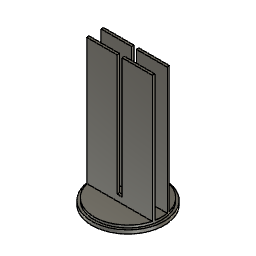
Can with 1 and 2 Vertical Shelves (Autodesk Fusion 360 design; units mm, degrees)
Autodesk Fusion 360 part; units mm, degrees
sketch "Base" plane through (0, 0, 0) normal (0, 0, 1) x (1, 0, 0)
  circle A0 centre (0, 0) radius 30
  circle A1 centre (0, 0) radius 28
  dimension "d1" = 60
  dimension "d2" = 56
  constraint coincident A0.centre A1.centre
  constraint concentric A0 A1
  measures "d1" diameter of A0
  measures "d2" diameter of A1
extrude "Extrude1" add sketch "Base" along normal blind 2 contours A1 makes body 1
extrude "Extrude2" add sketch "Base" along normal blind 113 bodies 1
sketch "Sketch2" plane through (0, 0, 0) normal (0, 0, 1) x (1, 0, 0)
  circle A0 centre (0, 0) radius 28
  line L0 (0, -2) -> (27.9285, -2)
  line L1 (-27.9285, -2) -> (0, -2)
  line L2 (0, 2) -> (-27.9285, 2)
  line L3 (27.9285, 2) -> (0, 2)
  circle A1 centre (0, 0) radius 30
  constraint coincident A0.centre A1.centre
  constraint coincident A0 L0.end
  constraint horizontal L0
  constraint coincident A0 L1.start
  constraint parallel L0 L1
  constraint coincident A0 L2.end
  constraint parallel L0 L2
  constraint coincident A0 L3.start
  constraint parallel L2 L3
extrude "Extrude3" add sketch "Sketch2" along normal blind 3 separate body makes body 2
extrude "Extrude4" add sketch "Sketch2" along normal blind 5 contours A0 L0 L1 bodies 2
extrude "Extrude5" add sketch "Sketch2" along normal blind 5 contours A0 L2 L3 bodies 2
extrude "Extrude6" add sketch "Sketch2" along normal blind 110 contours A0 L0 L1 L2 L3 bodies 2
sketch "Sketch6" plane through (0, 2, 0) normal (0, 1, 0) x (-1, 0, 0)
  line L0 (-27.9285, 5) -> (27.9285, 5)
  line L1 (27.9285, 5) -> (27.9285, 110)
  line L2 (27.9285, 110) -> (-27.9285, 110)
  line L3 (-27.9285, 110) -> (-27.9285, 5)
  line L4 (-2.5, 7.5) -> (2.5, 7.5)
  line L5 (2.5, 7.5) -> (2.5, 110)
  line L6 (-2.5, 110) -> (2.5, 110)
  line L7 (-2.5, 110) -> (-2.5, 7.5)
  dimension "d15" = 102.5
  dimension "d16" = 5
  constraint parallel L0 L4
  constraint coincident L2 L5.end
  constraint perpendicular L2 L5
  constraint coincident L2 L6.start
  constraint perpendicular L4 L7
  measures "d15" distance of L4.end L5.end
  measures "d16" distance of L5.end L6.start
extrude "Extrude7" cut sketch "Sketch6" against normal blind 4 contours L2 L4 L5 L6 L7 bodies 2
sketch "Sketch7" plane through (0, 0, 0) normal (0, 0, 1) x (1, 0, 0)
  circle A0 centre (-100, 0) radius 30
  circle A1 centre (-100, 0) radius 28
  line L0 (-100, 5) -> (-72.45, 5)
  line L1 (-100, -5) -> (-72.45, -5)
  line L2 (-100, -5) -> (-127.55, -5)
  line L3 (-100, 5) -> (-127.55, 5)
  line L4 (-100, -7) -> (-72.8891, -7)
  line L5 (-100, -7) -> (-127.1109, -7)
  line L6 (-100, 7) -> (-72.8891, 7)
  line L7 (-100, 7) -> (-127.1109, 7)
  constraint coincident A1 L0.end
  constraint coincident A1 L1.end
  constraint coincident A1 L2.end
  constraint coincident A1 L3.end
  constraint coincident A1 L4.end
  constraint parallel L2 L4
  constraint coincident A1 L5.end
  constraint parallel L4 L5
  constraint coincident A1 L6.end
  constraint horizontal L6
  constraint coincident A1 L7.end
  constraint parallel L6 L7
extrude "Extrude8" add sketch "Sketch7" along normal blind 3 separate body makes body 3
extrude "Extrude9" add sketch "Sketch7" along normal blind 5 contours A1 L6 L7 bodies 3
extrude "Extrude10" add sketch "Sketch7" along normal blind 5 contours A1 L0 L1 L2 L3 bodies 3
extrude "Extrude11" add sketch "Sketch7" along normal blind 5 contours A1 L4 L5 bodies 3
extrude "Extrude12" add sketch "Sketch7" along normal blind 110 contours A1 L0 L3 L6 L7 bodies 3
extrude "Extrude13" add sketch "Sketch7" along normal blind 110 contours A1 L1 L2 L4 L5 bodies 3
sketch "Sketch8" plane through (0, -7, 0) normal (0, -1, 0) x (1, 0, 0)
  line L0 (-127.1109, 5) -> (-72.8891, 5)
  line L1 (-72.8891, 5) -> (-72.8891, 110)
  line L2 (-72.8891, 110) -> (-127.1109, 110)
  line L3 (-127.1109, 110) -> (-127.1109, 5)
  line L4 (-102, 10) -> (-98, 10)
  line L5 (-98, 10) -> (-98, 110)
  line L6 (-102, 10) -> (-102, 110)
  constraint horizontal L4
  constraint coincident L2 L5.end
  constraint perpendicular L2 L5
  constraint coincident L2 L6.end
  constraint perpendicular L2 L6
extrude "Extrude14" cut sketch "Sketch8" against normal blind 200 contours L2 L4 L5 L6 bodies 3
hidden bodies 1 2
named bodies: "Bottom"
